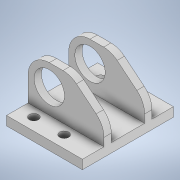
# Autodesk Inventor part: beslag_board_3D
Saved by Autodesk Inventor 2022 (Build 260153000, 153)
## iProperties
Created: 2022-04-10
Part Number: beslag_board_3D
Material: Generic
Document SubType Name: Modeling
Designer: Patrick
Density: 1 g/cm^3
Appearance: Default
Author: Patrick
Autodesk Inventor part; units mm, degrees
ref_plane "YZ Plane" through (0, 0, 0) normal (1, 0, 0) x (0, 1, 0)
ref_plane "XZ Plane" through (0, 0, 0) normal (0, 1, 0) x (-1, 0, 0)
ref_plane "XY Plane" through (0, 0, 0) normal (0, 0, 1) x (1, 0, 0)
sketch "Sketch1" plane through (0, 0, 0) normal (0, 1, 0) x (-1, 0, 0)
  line L0 (0, 0) -> (25, 0)
  line L1 (25, 0) -> (25, -30)
  line L2 (25, -30) -> (0, -30)
  line L3 (0, -30) -> (0, 0)
  circle A0 centre (20, -4) radius 1.5
  circle A1 centre (20, -26) radius 1.5
  circle A2 centre (10, -4) radius 1.5
  circle A3 centre (10, -26) radius 1.5
  dimension "d0" = 30
  dimension "d1" = 25
  dimension "d2" = 3
  dimension "d5" = 22
  dimension "d8" = 10
  dimension "d11" = 20
  dimension "d12" = 4
  constraints: 8 end point, 4 centre point, 2 horizontal, 2 parallel, 1 perpendicular, 1 vertical, 6 other
  measures "d0" distance of L2.end L0.start
  measures "d1" distance of L1.end L2.end
  measures "d2" diameter of A0
  measures "d5" distance of A0.centre A1.centre
  measures "d8" distance of A0.centre A2.centre
  measures "d11" distance from line of A0.centre L3
  measures "d12" distance from line of L0 A0.centre
extrude "Extrusion1" add sketch "Sketch1" along normal blind 25.5
sketch "Sketch2" plane through (0, 0, 0) normal (1, 0, 0) x (0, 0, -1)
  line L0 (0, 0) -> (30, 0) projected
  line L1 (30, 0) -> (30, 25.5) projected
  line L2 (0, 25.5) -> (30, 25.5) projected
  line L3 (0, 0) -> (0, 25.5) projected
  line L4 (9.5, 25.5) -> (20.5, 25.5)
  line L5 (20.5, 25.5) -> (20.5, 3)
  line L6 (20.5, 3) -> (9.5, 3)
  line L7 (9.5, 3) -> (9.5, 25.5)
  line L8 (30, 25.5) -> (0, 25.5) projected
  line L9 (30, 0) -> (30, 25.5) projected
  line L10 (22.9, 25.5) -> (30, 25.5)
  line L11 (30, 25.5) -> (30, 3)
  line L12 (30, 3) -> (22.9, 3)
  line L13 (22.9, 3) -> (22.9, 25.5)
  line L14 (0, 25.5) -> (7.1, 25.5)
  line L15 (7.1, 25.5) -> (7.1, 3)
  line L16 (7.1, 3) -> (0, 3)
  line L17 (0, 3) -> (0, 25.5)
  point P0 (0, 3)
  point P1 (30, 3)
  dimension "d15" = 3
  dimension "d16" = 3
  dimension "d17" = 3
  dimension "d19" = 11
  dimension "d20" = 2.4
  dimension "d21" = 2.4
  dimension "d22" = 7.1
  constraints: 24 end point, 6 parallel, 3 horizontal, 3 perpendicular, 3 point on line
  measures "d15" distance between parallel lines of L0 L16
  measures "d16" distance between parallel lines of L0 L12
  measures "d17" distance between parallel lines of L0 L6
  measures "d19" distance between parallel lines of L7 L5
  measures "d20" distance between parallel lines of L13 L5
  measures "d21" distance between parallel lines of L15 L7
  measures "d22" distance between parallel lines of L13 L1
extrude "Extrusion2" cut sketch "Sketch2" against normal blind 25.5 contours L3 L2 L15 L16 | L12 L13 L2 L1 | L2 L5 L6 L7
sketch "Sketch3" plane through (0, 3, -7.1) normal (0, 0, 1) x (1, 0, 0)
  circle A0 centre (-18, 8) radius 5
  line L0 (-25, 0) -> (-25, 22.5) projected
  line L1 (0, 0) -> (-25, 0) projected
  line L2 (0, 22.5) -> (0, 0) projected
  line L3 (-25, 22.5) -> (0, 22.5) projected
  line L4 (-25, 15) -> (-11, 15)
  line L5 (-11, 15) -> (0, 6)
  line L6 (0, 0) -> (0, 22.5) projected
  point P0 (0, -3)
  point P1 (0, 6)
  dimension "d25" = 8
  dimension "d26" = 7
  dimension "d27" = 7
  dimension "d28" = 14
  dimension "d29" = 6
  dimension "d30" = 10
  constraints: 4 end point, 2 point on line, 1 centre point, 1 horizontal
  measures "d25" distance from line of L1 A0.centre
  measures "d26" distance from line of L0 A0.centre
  measures "d27" distance from line of L4 A0.centre
  measures "d28" distance of L4.start L4.end
  measures "d29" distance from line of L1 L5.end
  measures "d30" diameter of A0
extrude "Extrusion3" cut sketch "Sketch3" against normal blind 25.5 contours A0 | L0 L3 L2 L5 L4
fillet "Fillet1" radius 7 6 edges at (-25, 18, -21.7) (-11, 18, -21.7) (0, 9, -21.7) (-11, 18, -8.3) (0, 9, -8.3) (-25, 18, -8.3)
body "Solid1"
